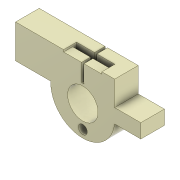
# Autodesk Inventor part: Prowadnica_tloka
Saved by Autodesk Inventor 2021 (Build 250183000, 183)
## iProperties
Created: 2022-10-06
Part Number: Prowadnica_tloka
Material: PC/ABS Plastic
Document SubType Name: Modeling
Designer: agnpi
Density: 0.357273 g/cm^3
Appearance: Smooth - Ash
Author: agnpi
Autodesk Inventor part; units mm, degrees
ref_plane "YZ Plane" through (0, 0, 0) normal (1, 0, 0) x (0, 1, 0)
ref_plane "XZ Plane" through (0, 0, 0) normal (0, 1, 0) x (-1, 0, 0)
ref_plane "XY Plane" through (0, 0, 0) normal (0, 0, 1) x (1, 0, 0)
sketch "Sketch1" plane through (0, 0, 0) normal (0, 0, 1) x (1, 0, 0)
  circle A0 centre (0, 0.75) radius 6.45
  circle A1 centre (0, -8.775) radius 1.9
  line L0 (-18.9, 0) -> (18.9, 0) construction
  line L1 (0, -17.6918) -> (0, 22.1508) construction
  line L2 (-0.5, 16.459) -> (-0.5, 8.23)
  line L3 (-0.5, 8.23) -> (0.5, 8.23)
  line L4 (0.5, 8.23) -> (0.5, 16.4588)
  line L5 (-12.7, 16.459) -> (-0.5, 16.459)
  line L6 (0.5, 16.4588) -> (12.7, 16.4588)
  line L7 (-12.7, 16.459) -> (-13.5, 16.459)
  line L8 (12.7, 16.4588) -> (13.5, 16.4588)
  line L9 (13.5, 16.4588) -> (13.5, 0)
  line L10 (-13.5, 16.459) -> (-13.5, 0)
  arc A2 (-13.5, 0) -> (13.5, 0) centre (0, 1.5937) ccw
  dimension "d0" = 12.9
  dimension "d1" = 3.8
  dimension "d11" = 1
  dimension "d33" = 0.8
  dimension "d34" = 0.8
  dimension "d35" = 27
  dimension "d36" = 13
  dimension "d37" = 13.5
  dimension "d40" = 15.709
  dimension "d44" = 13.5938
  dimension "d45" = 9.525
  dimension "d47" = 15.7088
  dimension "d54" = 7.48
  dimension "d55" = 6.6363
  constraints: 18 end point, 5 perpendicular, 4 horizontal, 4 point on line, 3 centre point, 2 point on circle, 1 vertical
  measures "d0" diameter of A0
  measures "d1" diameter of A1
  measures "d11" distance of L2.end L3.end
  measures "d33" distance of L5.start L7.end
  measures "d34" distance of L6.end L8.end
  measures "d35" distance of L8.end L7.end
  measures "d36" distance between parallel lines of L9 L4
  measures "d37" distance between parallel lines of L1 L10
  measures "d40" distance from line of A0.centre L5
  measures "d44" radius of A2
  measures "d45" distance of A0.centre A1.centre
  measures "d47" distance from line of L6 A0.centre
  measures "d54" distance from line of A0.centre L3
  measures "d55" vertical distance of L2.end A2.centre
extrude "Extrusion1" add sketch "Sketch1" along normal blind 10
sketch "Sketch2" plane through (0.5, 16.4588, 0) normal (0, 1, 0) x (1, 0, 0)
  line L0 (0, 0) -> (0, -10) projected
  line L1 (0, -10) -> (7.63, -10)
  line L2 (7.63, -10) -> (7.63, -6.2)
  line L3 (7.63, -6.2) -> (0, -6.2)
  line L4 (0, -6.2) -> (0, -10)
  line L5 (-1, -10) -> (-14, -10) projected
  line L6 (-1, -10) -> (-8.63, -10)
  line L7 (-8.63, -10) -> (-8.63, -6.2)
  line L8 (-8.63, -6.2) -> (-1, -6.2)
  line L9 (-1, -6.2) -> (-1, -10)
  line L10 (-8.63, -6.2) -> (7.63, -6.2)
  line L11 (7.63, -6.2) -> (7.63, -4.5)
  line L12 (7.63, -4.5) -> (-8.63, -4.5)
  line L13 (-8.63, -4.5) -> (-8.63, -6.2)
  point P0 (-0.5, 0)
  point P1 (-13.2, -10)
  point P2 (7.63, -6.2)
  point P3 (-8.63, -10)
  dimension "d18" = 7.63
  dimension "d19" = 3.8
  dimension "d20" = 7.63
  dimension "d21" = 3.8
  dimension "d22" = 1.7
  constraints: 24 end point, 6 parallel, 3 horizontal, 3 perpendicular, 1 collinear
  measures "d18" distance of L3.end L2.end
  measures "d19" distance of L2.end L1.end
  measures "d20" distance of L7.end L8.end
  measures "d21" distance of L6.end L7.end
  measures "d22" distance of L11.end L10.end
extrude "Extrusion2" cut sketch "Sketch2" against normal blind 8 contours L10 L8 L13 L12 L0 | L0 L12 L11 L3
extrude "Extrusion3" cut sketch "Sketch2" against normal blind 0.85 contours L3 L2 L1 L0 | L9 L5 L7 L8
sketch "Sketch4" plane through (13.5, 0, 0) normal (1, 0, 0) x (0, 0, -1)
  line L0 (0, 0) -> (-10, 0) projected
  line L1 (0, 0) -> (0, 16.4588) projected
  line L2 (-10, 0) -> (0, 0)
  line L3 (0, 0) -> (0, 6)
  line L4 (0, 6) -> (-10, 6)
  line L5 (-10, 6) -> (-10, 0)
  dimension "d56" = 6
  constraints: 8 end point, 2 parallel, 1 horizontal, 1 perpendicular, 1 point on line
  measures "d56" distance of L3.end L2.end
extrude "Extrusion5" add sketch "Sketch4" along normal blind 11.11
sketch "Sketch5" plane through (-13.5, 16.459, 0) normal (0, 1, 0) x (1, 0, 0)
  point P0 (13.5, 0)
sketch "Sketch6" plane through (-13.5, 16.459, 0) normal (0, 1, 0) x (1, 0, 0)
  line L0 (5.37, -6.2) -> (5.37, -4.5) projected
  line L1 (13, 0) -> (13, -10) projected
  line L2 (5.37, -6.2) -> (13, -6.2)
  line L3 (13, -6.2) -> (13, -10)
  line L4 (13, -10) -> (5.37, -10)
  line L5 (5.37, -10) -> (5.37, -6.2)
  line L6 (5.37, -4.5) -> (13, -4.5) projected
  line L7 (5.37, -6.2) -> (13, -6.2)
  line L8 (13, -6.2) -> (13, -4.5)
  line L9 (13, -4.5) -> (5.37, -4.5)
  line L10 (5.37, -4.5) -> (5.37, -6.2)
  point P0 (13.5, 0)
  constraints: 16 end point, 4 parallel, 2 horizontal, 2 perpendicular
extrude "Extrusion6" cut sketch "Sketch6" against normal up to surface (0.8502 mm away) contours L2 L1 L4 L5
extrude "Extrusion7" cut sketch "Sketch6" against normal blind 8 contours L0 L6 L1 L2
sketch "Sketch7" plane through (-13.5, 0, 0) normal (-1, 0, 0) x (0, 0, 1)
  line L0 (0, 16.459) -> (10, 16.459) projected
  line L1 (10, 16.459) -> (10, 0) projected
  line L2 (0, 16.459) -> (10, 16.459)
  line L3 (10, 16.459) -> (10, 9.159)
  line L4 (10, 9.159) -> (0, 9.159)
  line L5 (0, 9.159) -> (0, 16.459)
  point P0 (0, 0)
  dimension "d63" = 7.3
  constraints: 8 end point, 2 parallel, 1 horizontal, 1 perpendicular, 1 point on line
  measures "d63" distance of L2.end L3.end
extrude "Extrusion8" add sketch "Sketch7" along normal blind 14
sketch "Sketch8" plane through (-13.5, 9.159, 0) normal (0, -1, 0) x (1, 0, 0)
  line L0 (13, 0) -> (-14, 0) projected
  line L1 (27, 10) -> (0, 10) projected
  line L2 (-14, 0) -> (0, 0)
  line L3 (0, 0) -> (0, 10)
  line L4 (0, 10) -> (-14, 10)
  line L5 (-14, 10) -> (-14, 0)
  point P0 (13.5, 0)
  constraints: 8 end point, 2 parallel, 1 horizontal, 1 perpendicular
extrude "Extrusion9" add sketch "Sketch8" along normal blind 7
move faces "Move1" translate (-1, 0, 0) faces at (-27.5, 11.6923, 6.6667)
body "Solid1"
